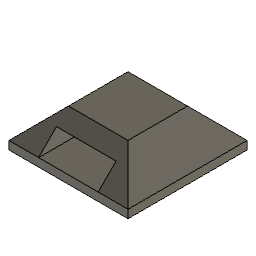
Kabelbinderhalter (Autodesk Fusion 360 design; units mm, degrees)
part number: 2025-12-09-21-00-14-927
Autodesk Fusion 360 part; units mm, degrees
sketch "Skizze1" plane through (0, 0, 0) normal (0, 0, 1) x (1, 0, 0)
  line L0 (0, 0) -> (20, 0)
  line L1 (20, 0) -> (20, 20)
  line L2 (20, 20) -> (0, 20)
  line L3 (0, 20) -> (0, 0)
  dimension "d1" = 20
  dimension "d2" = 20
  constraint horizontal L0
  constraint vertical L1
  constraint horizontal L2
  constraint vertical L3
  constraint coincident L0.start L3.end
  measures "d1" distance of L0.start L0.end
  measures "d2" distance of L0.start L2.end
extrude "Extrusion1" add sketch "Skizze1" along normal blind 1.4
sketch "Skizze2" plane through (0, 0, 1.4) normal (0, 0, 1) x (-1, 0, 0)
  line L0 (0, -20) -> (0, 0)
  line L1 (0, 0) -> (-20, 0)
  line L2 (-20, 0) -> (-20, -20)
  line L3 (-20, -20) -> (0, -20)
  line L4 (-15, -15) -> (-5, -15)
  line L5 (-5, -15) -> (-5, -5)
  line L6 (-5, -5) -> (-15, -5)
  line L7 (-15, -5) -> (-15, -15)
  line L8 (-15, -15) -> (-5, -5) construction
  line L9 (-5, -15) -> (-15, -5) construction
  point P0 (-10, -10)
  constraint horizontal L4
  constraint perpendicular L4 L5
  constraint parallel L4 L6
  constraint parallel L5 L7
  constraint coincident L8 P0
  constraint coincident L9 P0
extrude "Extrusion2" add sketch "Skizze2" along normal blind 5 contours L4 L5 L6 L7
chamfer "Fase1" distance 5 angle 45 4 edges at (10, 5, 1.4) (5, 10, 1.4) (10, 15, 1.4) (15, 10, 1.4)
sketch "Skizze3" plane through (0, 0, 0) normal (0, 1, 0) x (1, 0, 0)
  line L0 (0, 0) -> (0, -1.4)
  line L1 (0, -1.4) -> (20, -1.4)
  line L2 (10, -1.4) -> (10, -4.4)
  line L3 (10, -4.4) -> (7, -4.4)
  line L4 (7, -4.4) -> (13, -4.4)
  line L5 (13, -4.4) -> (13, -1.4)
  line L6 (13, -1.4) -> (7, -1.4)
  line L7 (7, -1.4) -> (7, -4.4)
  line L8 (7, -4.4) -> (5, -4.4)
  line L9 (5, -4.4) -> (15, -4.4)
  line L10 (15, -4.4) -> (15, -1.4)
  line L11 (15, -1.4) -> (5, -1.4)
  line L12 (5, -1.4) -> (5, -4.4)
  dimension "d8" = 2
  constraint coincident L0.start origin
  constraint vertical L0
  constraint perpendicular L0 L1
  constraint midpoint L1 L2.start
  constraint perpendicular L1 L2
  constraint perpendicular L2 L3
  constraint horizontal L4
  constraint vertical L5
  constraint horizontal L6
  constraint vertical L7
  constraint coincident L1 L5.end
  constraint perpendicular L7 L8
  constraint horizontal L9
  constraint vertical L10
  constraint horizontal L11
  constraint vertical L12
  constraint coincident L1 L10.end
  measures "d8" distance of L3.end L8.end
extrude "Extrusion3" cut sketch "Skizze3" along normal blind 21
sketch "Skizze4" plane through (0, 0, 0) normal (1, 0, 0) x (0, 1, 0)
  line L0 (0, 0) -> (0, 1.4)
  line L1 (0, 1.4) -> (5, 1.4)
  line L2 (5, 1.4) -> (15, 1.4)
  line L3 (15, 1.4) -> (15, 4.4)
  line L4 (15, 4.4) -> (5, 4.4)
  line L5 (5, 4.4) -> (5, 1.4)
  dimension "d11" = 10
  dimension "d12" = 3
  constraint coincident L0.start origin
  constraint vertical L0
  constraint perpendicular L0 L1
  constraint horizontal L2
  constraint vertical L3
  constraint horizontal L4
  constraint vertical L5
  measures "d11" distance of L1.end L2.end
  measures "d12" distance of L1.end L4.end
